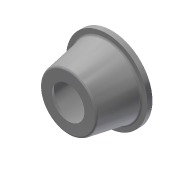
# Autodesk Inventor part: PP-08
Saved by Autodesk Inventor 2022 (Build 260148000, 148)
## iProperties
Created: 2008-09-23
Part Number: PP-08
Document SubType Name: Modeling
Designer: Mark Flayler
Mass: 0.0483679 g
Surface Area: 0.529275 cm^2
Volume: 0.00615368 cm^3
Density: 7.86 g/cm^3
Material: Steel, Mild
Description: DISPENSER RING
Appearance: Steel
Author: Mark Flayler
Autodesk Inventor part; units mm, degrees
ref_plane "YZ Plane" through (0, 0, 0) normal (1, 0, 0) x (0, 1, 0)
ref_plane "XZ Plane" through (0, 0, 0) normal (0, 1, 0) x (-1, 0, 0)
ref_plane "XY Plane" through (0, 0, 0) normal (0, 0, 1) x (1, 0, 0)
sketch "Sketch1" plane through (0, 0, 0) normal (0, 0, 1) x (1, 0, 0)
  line L0 (0, 0) -> (0, 2.15)
  line L1 (0.8, 0) -> (1.2969, 0)
  line L2 (1.3954, 0.0826) -> (1.7013, 1.8174)
  line L3 (1.7998, 1.9) -> (2, 1.9)
  line L4 (2, 1.9) -> (2, 2.15)
  line L5 (2, 2.15) -> (1.59, 2.15)
  line L6 (1.4915, 2.0674) -> (1.1856, 0.3326)
  line L7 (1.0872, 0.25) -> (0.95, 0.25)
  line L8 (0.95, 0.25) -> (0.8, 0)
  arc A0 (1.59, 2.15) -> (1.4915, 2.0674) centre (1.59, 2.05) ccw
  arc A1 (1.7998, 1.9) -> (1.7013, 1.8174) centre (1.7998, 1.8) ccw
  arc A2 (1.0872, 0.25) -> (1.1856, 0.3326) centre (1.0872, 0.35) ccw
  arc A3 (1.2969, 0) -> (1.3954, 0.0826) centre (1.2969, 0.1) ccw
  point P0 (1.5061, 2.15)
  dimension "d0" = 1.6
  dimension "d2" = 1.9
  dimension "d3" = 0.25
  dimension "d4" = 2.15
  dimension "d5" = 80
  dimension "d6" = 0.1
  dimension "d8" = 3.18
  dimension "d9" = 4
  dimension "d10" = 0.25
  dimension "d11" = 0.25
  dimension "d12" = 0.1
  constraints: 18 end point, 8 point on circle, 8 tangent, 4 centre point, 4 parallel, 2 equal radius, 2 horizontal alignment, 2 perpendicular, 2 point on line, 1 vertical
  measures "d0" diameter of L1.start L0
  measures "d2" diameter of L7.end L0
  measures "d3" distance between parallel lines of L1 L7
  measures "d4" distance from line of L0.start L5
  measures "d5" angle of L2 L1
  measures "d6" radius of A0
  measures "d8" diameter of A0.centre L0
  measures "d9" diameter of L4 L0
  measures "d10" distance between parallel lines of L2 L6
  measures "d11" distance between parallel lines of L5 L3
  measures "d12" radius of A1
revolve "Revolution1" add sketch "Sketch1" angle 360 about axis through (0, 0, 0) along (0, 1, 0)
body "Solid1"
